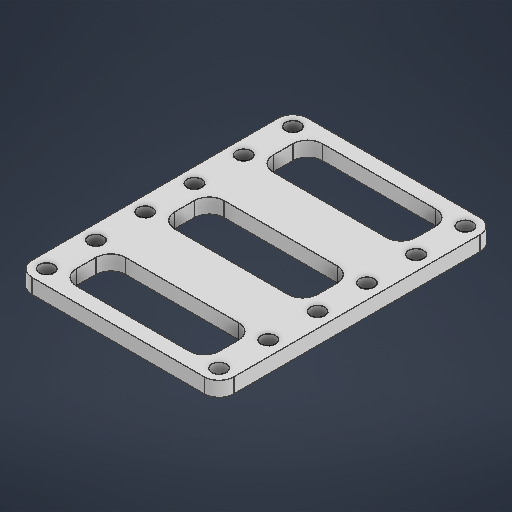
# Autodesk Inventor part: base_extender
Saved by Autodesk Inventor 2026.1 (Build 301233000, 233)
## iProperties
Created: 2026-01-07
Part Number: base_extender
Material: Generic
Document SubType Name: Modeling
Designer: emanuel
Density: 1 g/cm^3
Appearance: Default
Author: emanuel
Autodesk Inventor part; units mm, degrees
ref_plane "YZ Plane" through (0, 0, 0) normal (1, 0, 0) x (0, 1, 0)
ref_plane "XZ Plane" through (0, 0, 0) normal (0, 1, 0) x (-1, 0, 0)
ref_plane "XY Plane" through (0, 0, 0) normal (0, 0, 1) x (1, 0, 0)
sketch "Sketch1" plane through (0, 0, 0) normal (0, 1, 0) x (-1, 0, 0)
  line L0 (0, 0) -> (35, 0)
  line L1 (35, 0) -> (35, -50)
  line L2 (35, -50) -> (0, -50)
  line L3 (0, -50) -> (0, 0)
  line L4 (0, 0) -> (0, -10)
  line L5 (0, -10) -> (0, -20)
  line L6 (0, -20) -> (0, -30)
  line L7 (0, -30) -> (0, -40)
  line L8 (35, 0) -> (35, -10)
  line L9 (35, -10) -> (35, -20)
  line L10 (35, -20) -> (35, -30)
  line L11 (35, -30) -> (35, -40)
  circle A0 centre (35, 0) radius 1.5
  circle A1 centre (35, -10) radius 1.5
  circle A2 centre (35, -20) radius 1.5
  circle A3 centre (35, -30) radius 1.5
  circle A4 centre (35, -40) radius 1.5
  circle A5 centre (35, -50) radius 1.5
  circle A6 centre (0, -50) radius 1.5
  circle A7 centre (0, -40) radius 1.5
  circle A8 centre (0, -30) radius 1.5
  circle A9 centre (0, -20) radius 1.5
  circle A10 centre (0, -10) radius 1.5
  circle A11 centre (0, 0) radius 1.5
  line L12 (35, -50) -> (38, -50)
  line L13 (38, -50) -> (38, -53)
  line L14 (38, -53) -> (35, -53)
  line L15 (35, -53) -> (35, -50)
  line L16 (0, 0) -> (-3, 0)
  line L17 (-3, 0) -> (-3, 3)
  line L18 (-3, 3) -> (0, 3)
  line L19 (0, 3) -> (0, 0)
  line L20 (-3, 3) -> (38, 3)
  line L21 (38, 3) -> (38, -53)
  line L22 (38, -53) -> (-3, -53)
  line L23 (-3, -53) -> (-3, 3)
  line L24 (35, 0) -> (0, 0)
  line L25 (0, 0) -> (0, -10)
  line L26 (0, -10) -> (35, -10)
  line L27 (35, -10) -> (35, 0)
  line L28 (35, -10) -> (0, -10)
  line L29 (0, -10) -> (0, -20)
  line L30 (0, -20) -> (35, -20)
  line L31 (35, -20) -> (35, -10)
  line L32 (35, -20) -> (0, -20)
  line L33 (0, -20) -> (0, -30)
  line L34 (0, -30) -> (35, -30)
  line L35 (35, -30) -> (35, -20)
  line L36 (35, -30) -> (0, -30)
  line L37 (0, -30) -> (0, -40)
  line L38 (0, -40) -> (35, -40)
  line L39 (35, -40) -> (35, -30)
  line L40 (35, 0) -> (32, 0)
  line L41 (32, 0) -> (32, -50)
  line L42 (32, -50) -> (35, -50)
  line L43 (35, -50) -> (35, 0)
  line L44 (0, 0) -> (3, 0)
  line L45 (3, 0) -> (3, -50)
  line L46 (3, -50) -> (0, -50)
  line L47 (0, -50) -> (0, 0)
  point P0 (32, 0)
  point P1 (32, -10)
  point P2 (3, -10)
  point P3 (3, -40)
  point P4 (32, -40)
  point P5 (3, -20)
  point P6 (32, -20)
  point P7 (32, -30)
  point P8 (3, -30)
  dimension "d0" = 35
  dimension "d1" = 50
  dimension "d2" = 10
  dimension "d3" = 10
  dimension "d4" = 10
  dimension "d5" = 10
  dimension "d6" = 10
  dimension "d7" = 10
  dimension "d8" = 10
  dimension "d9" = 10
  dimension "d10" = 3
  dimension "d11" = 3
  dimension "d12" = 3
  dimension "d13" = 3
  dimension "d14" = 3
  dimension "d15" = 3
  dimension "d16" = 3
  dimension "d17" = 3
  dimension "d18" = 3
  dimension "d19" = 3
  dimension "d20" = 3
  dimension "d21" = 3
  dimension "d22" = 3
  dimension "d23" = 3
  dimension "d24" = 3
  dimension "d25" = 3
  dimension "d26" = 3
  dimension "d27" = 3
  constraints: 96 end point, 20 parallel, 12 centre point, 12 coincident, 10 horizontal, 10 perpendicular, 10 point on line
  measures "d0" distance of L1.end L2.end
  measures "d1" distance of L0.end L1.end
  measures "d2" distance of L0.start L4.end
  measures "d3" distance of L4.end L5.end
  measures "d4" distance of L5.end L6.end
  measures "d5" distance of L6.end L7.end
  measures "d6" distance of L0.end L8.end
  measures "d7" distance of L8.end L9.end
  measures "d8" distance of L9.end L10.end
  measures "d9" distance of L10.end L11.end
  measures "d10" diameter of A0
  measures "d11" diameter of A1
  measures "d12" diameter of A2
  measures "d13" diameter of A3
  measures "d14" diameter of A4
  measures "d15" diameter of A5
  measures "d16" diameter of A6
  measures "d17" diameter of A7
  measures "d18" diameter of A8
  measures "d19" diameter of A9
  measures "d20" diameter of A10
  measures "d21" diameter of A11
  measures "d22" distance of L13.end L14.end
  measures "d23" distance of L12.end L13.end
  measures "d24" distance of L17.end L18.end
  measures "d25" distance of L16.end L17.end
  measures "d26" distance of L42.end L41.end
  measures "d27" distance of L45.end L46.end
extrude "Extrusion1" add sketch "Sketch1" along normal blind 3 contours A11 L19 L20 L21 L12 A5 L1 A4 A3 A2 A1 A0 L0 | L0 L45 L26 A10 L3 A11 | L3 A10 A9 A8 A7 A6 L2 A5 L15 L22 L23 L16 A11 | L16 L17 L18 L19 A11 | L0 A0 L1 A1 L26 L41 | L45 L30 A9 L3 A10 L26 | L26 L41 L30 L45 | L26 A1 L1 A2 L30 L41 | L45 L34 A8 L3 A9 L30 | L15 A5 L12 L13 L14 | L30 A2 L1 A3 L34 L41 | L45 L38 A7 L3 A8 L34 | L34 L41 L38 L45 | L34 A3 L1 A4 L38 L41 | L45 L2 A6 L3 A7 L38 | L2 L41 L38 A4 L1 A5
fillet "Fillet1" radius 3 16 edges at (3, 1.5, 3) (-38, 1.5, 3) (-38, 1.5, -53) (3, 1.5, -53) (-32, 1.5, -50) (-32, 1.5, -40) (-3, 1.5, -40) (-3, 1.5, -50) (-3, 1.5, -30) (-3, 1.5, -20) (-32, 1.5, -20) (-32, 1.5, -30) (-32, 1.5, -10) (-32, 1.5, 0) (-3, 1.5, 0) (-3, 1.5, -10)
body "Solid1"
